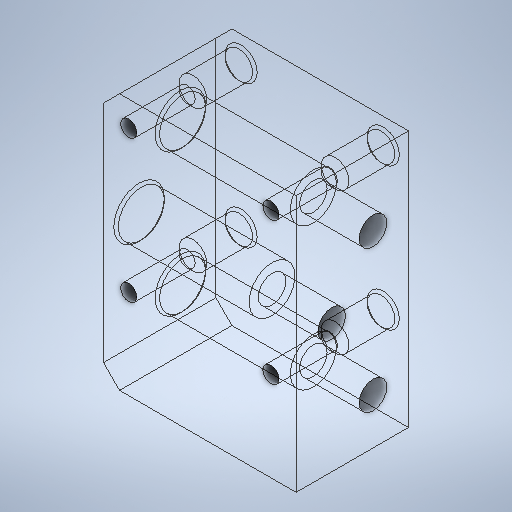
# Autodesk Inventor part: ZaxisMotorMount
Saved by Autodesk Inventor 2025.1 (Build 291241000, 241)
## iProperties
Created: 2024-10-09
Part Number: ZaxisMotorMount
Material: Generic
Document SubType Name: Modeling
Designer: maxda
Density: 1 g/cm^3
Appearance: Default
Author: maxda
## iProperties of the stored document ZaxisMotorMount_3DPrint.ipt
Created: 2024-10-09
Part Number: ZaxisMotorMount_3DPrint
Material: Generic
Document SubType Name: Modeling
Designer: maxda
Density: 1 g/cm^3
Appearance: Default
Author: maxda
Autodesk Inventor part; units mm, degrees
ref_plane "YZ Plane" through (0, 0, 0) normal (1, 0, 0) x (0, 1, 0)
ref_plane "XZ Plane" through (0, 0, 0) normal (0, 1, 0) x (-1, 0, 0)
ref_plane "XY Plane" through (0, 0, 0) normal (0, 0, 1) x (1, 0, 0)
sketch "Sketch1" plane through (0, 0, 0) normal (1, 0, 0) x (0, 1, 0)
  line L0 (-28, 12.25) -> (28, 12.25)
  line L1 (28, 12.25) -> (28, -12.25)
  line L2 (28, -12.25) -> (-28, -12.25)
  line L3 (-28, -12.25) -> (-28, 12.25)
  line L4 (-28, 12.25) -> (28, -12.25) construction
  line L5 (28, 12.25) -> (-28, -12.25) construction
  circle A0 centre (13, -4.5) radius 5
  circle A1 centre (0, 4.5) radius 5
  circle A2 centre (-18, -4.5) radius 5
  circle A3 centre (13, -4.5) radius 3
  circle A4 centre (0, 4.5) radius 3
  circle A5 centre (-18, -4.5) radius 3
  point P0 (0, 0)
  dimension "d2" = 56
  dimension "d3" = 24.5
  dimension "d4" = 10
  dimension "d5" = 4.5
  dimension "d6" = 4.5
  dimension "d7" = 15
  dimension "d8" = 6
  dimension "d27" = 10
  constraints: 12 end point, 6 centre point, 4 equal radius, 3 coincident, 2 midpoint, 2 parallel, 1 horizontal, 1 horizontal alignment, 1 perpendicular, 1 vertical alignment
  measures "d2" distance between parallel lines of L1 L3
  measures "d3" distance between parallel lines of L0 L2
  measures "d4" diameter of A1
  measures "d5" distance of A1.centre point (0, 0)
  measures "d6" vertical distance of A0.centre point (0, 0)
  measures "d7" distance from line of L1 A0.centre
  measures "d8" diameter of A4
  measures "d27" distance from line of L3 A2.centre
extrude "Extrusion1" add sketch "Sketch1" along normal blind 42 contours L0 L1 L2 L3 | A0 | A1 | A2
extrude "Extrusion2" cut sketch "Sketch1" along normal blind 29 contours A0 | A1 | A2
sketch "Sketch2" plane through (0, -28, 12.25) normal (0, 0, 1) x (1, 0, 0)
  circle A0 centre (5.5, 50.5) radius 1.75
  circle A1 centre (36.5, 50.5) radius 1.75
  circle A2 centre (36.5, 19.5) radius 1.75
  circle A3 centre (5.5, 19.5) radius 1.75
  line L0 (0, 56) -> (42, 56) projected
  line L1 (0, 56) -> (0, 0) projected
  circle A4 centre (36.5, 50.5) radius 3
  circle A5 centre (5.5, 50.5) radius 3
  circle A6 centre (5.5, 19.5) radius 3
  circle A7 centre (36.5, 19.5) radius 3
  point P0 (0, 28)
  dimension "d11" = 5.5
  dimension "d12" = 5.5
  dimension "d13" = 31
  dimension "d14" = 31
  dimension "d15" = 3.5
  dimension "d21" = 6
  constraints: 8 centre point, 6 equal radius, 4 coincident, 2 horizontal alignment, 2 vertical alignment
  measures "d11" distance from line of L0 A0.centre
  measures "d12" distance from line of L1 A0.centre
  measures "d13" distance of A1.centre A0.centre
  measures "d14" distance of A2.centre A1.centre
  measures "d15" diameter of A0
  measures "d21" diameter of A5
extrude "Extrusion3" cut sketch "Sketch2" against normal blind 28.75 contours A0 | A1 | A2 | A3
chamfer "Chamfer1" distance 3.5 angle 45 2 edges at (0, 28, 0) (0, -28, 0)
sketch "Sketch3" plane through (42, -28, -12.25) normal (0, 0, -1) x (-1, 0, 0)
  circle A0 centre (5.5, 50.5) radius 3 projected
  circle A1 centre (36.5, 50.5) radius 3 projected
  circle A2 centre (36.5, 19.5) radius 3 projected
  circle A3 centre (5.5, 19.5) radius 3 projected
  point P0 (42, 28)
extrude "Extrusion4" cut sketch "Sketch3" against normal blind 10.5
chamfer "Chamfer2" distance 1.25 angle 45 4 edges at (34.75, 22.5, -1.75) (3.75, 22.5, -1.75) (3.75, -8.5, -1.75) (34.75, -8.5, -1.75)
chamfer "Chamfer3" distance 0.5 angle 45 7 edges at (39.5, 22.5, -12.25) (8.5, 22.5, -12.25) (0, 8, -4.5) (0, -5, 4.5) (0, -23, -4.5) (8.5, -8.5, -12.25) (39.5, -8.5, -12.25)
body "Solid1"
